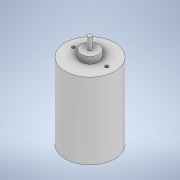
# Autodesk Inventor part: Helion_Motor
Saved by Autodesk Inventor 2022.3 (Build 263350000, 350)
## iProperties
Created: 2022-05-19
Part Number: Helion_Motor
Material: Generic
Document SubType Name: Modeling
Designer: Mlees
Density: 1 g/cm^3
Appearance: Default
Author: Mlees
Autodesk Inventor part; units mm, degrees
ref_plane "YZ Plane" through (0, 0, 0) normal (1, 0, 0) x (0, 1, 0)
ref_plane "XZ Plane" through (0, 0, 0) normal (0, 1, 0) x (-1, 0, 0)
ref_plane "XY Plane" through (0, 0, 0) normal (0, 0, 1) x (1, 0, 0)
sketch "Sketch1" plane through (0, 0, 0) normal (0, 1, 0) x (-1, 0, 0)
  circle A0 centre (0, 0) radius 18.625
  dimension "d0" = 37.25
  constraints: 1 centre point, 1 coincident
  measures "d0" diameter of A0
extrude "Extrusion1" add sketch "Sketch1" along normal blind 57
sketch "Sketch2" plane through (0, 57, 0) normal (0, 1, 0) x (1, 0, 0)
  circle A0 centre (0, 0) radius 6.625
  dimension "d3" = 13.25
  constraints: 1 centre point, 1 coincident
  measures "d3" diameter of A0
extrude "Extrusion2" add sketch "Sketch2" along normal blind 5
sketch "Sketch3" plane through (0, 62, 0) normal (0, 1, 0) x (1, 0, 0)
  circle A0 centre (0, 0) radius 1.625
  dimension "d6" = 3.25
  constraints: 1 centre point, 1 coincident
  measures "d6" diameter of A0
extrude "Extrusion3" add sketch "Sketch3" along normal blind 9
sketch "Sketch4" plane through (0, 71, 0) normal (0, 1, 0) x (1, 0, 0)
  circle A0 centre (0, 0) radius 1.625 projected
  line L0 (0, 0.875) -> (-1.3693, 0.875)
  line L1 (0, 0.875) -> (1.3693, 0.875)
  arc A1 (1.3693, 0.875) -> (-1.3693, 0.875) centre (0, 0) ccw
  constraints: 4 end point, 4 point on circle, 2 horizontal, 1 centre point, 1 coincident, 1 concentric
extrude "Extrusion4" cut sketch "Sketch4" against normal blind 8 contours L1 L0 A0 picked at (0.8372, 0.9686)
sketch "Sketch5" plane through (0, 57, 0) normal (0, 1, 0) x (1, 0, 0)
  circle A0 centre (12.5, 0) radius 1.25
  circle A1 centre (-12.5, 0) radius 1.25
  line L0 (-12.5, 0) -> (0, 0)
  line L1 (0, 0) -> (12.5, 0)
  dimension "d13" = 2.5
  dimension "d14" = 2.5
  dimension "d17" = 12.5
  dimension "d18" = 12.5
  constraints: 4 end point, 2 centre point, 1 collinear, 1 horizontal
  measures "d13" diameter of A0
  measures "d14" diameter of A1
  measures "d17" distance of L0.end L1.end
  measures "d18" distance of L0.start L0.end
extrude "Extrusion5" cut sketch "Sketch5" against normal blind 8
body "Solid1"
